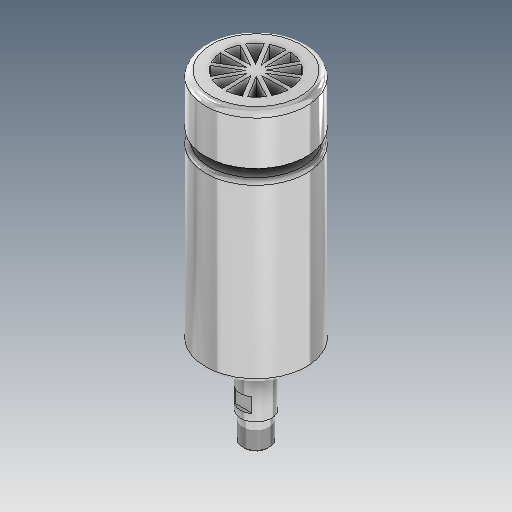
# Autodesk Inventor part: motor DC
Saved by Autodesk Inventor 2020 (Build 240168000, 168)
## iProperties
Created: 2020-05-03
Part Number: motor DC
Material: Genérico
Document SubType Name: Modeling
Designer: Leon
Density: 1 g/cm^3
Appearance: Cromo - Pulido
Mass: 286.743 g
Surface Area: 284.251 cm^2
Volume: 286.743 cm^3
Author: Leon
Autodesk Inventor part; units mm, degrees
ref_plane "YZ Plane" through (0, 0, 0) normal (1, 0, 0) x (0, 1, 0)
sketch "Boceto1" plane through (0, 0, 0) normal (0, 1, 0) x (-1, 0, 0)
  line L0 (66.6115, -79.4796) -> (66.6115, 152.1717)
  line L1 (66.6115, -79.4796) -> (92.6115, -79.4796)
  line L2 (92.6115, -79.4796) -> (92.6115, -53.9796)
  line L3 (92.6115, -53.9796) -> (79.6115, -53.9796)
  line L4 (79.6115, -53.9796) -> (79.6115, -48.4796)
  line L5 (79.6115, -48.4796) -> (92.6115, -48.4796)
  line L6 (92.6115, -48.4796) -> (92.6115, 41.8204)
  line L7 (92.6115, 41.8204) -> (79.6115, 41.8204)
  line L8 (79.6115, 41.8204) -> (79.6115, 48.3204)
  line L9 (79.6115, 48.3204) -> (70.6115, 48.3204)
  line L10 (70.6115, 48.3204) -> (70.6115, 51.8204)
  line L11 (70.6115, 51.8204) -> (74.6115, 51.8204)
  line L12 (74.6115, 51.8204) -> (74.6115, 71.8204)
  line L13 (74.6115, 71.8204) -> (73.5115, 71.8204)
  line L14 (73.5115, 71.8204) -> (73.5115, 86.3204)
  line L15 (73.5115, 86.3204) -> (66.6115, 86.3204)
  dimension "d8" = 26
  dimension "d9" = 25.5
  dimension "d10" = 13
  dimension "d11" = 5.5
  dimension "d12" = 90.3
  dimension "d20" = 13
  dimension "d21" = 6.5
  dimension "d22" = 9
  dimension "d23" = 3.5
  dimension "d24" = 4
  dimension "d25" = 20
  dimension "d26" = 1.1
  dimension "d27" = 14.5
  constraints: 32 end point, 10 perpendicular, 3 horizontal, 3 vertical, 2 point on line
  measures "d8" distance of L0.start L1.end
  measures "d9" distance of L1.end L2.end
  measures "d10" distance of L2.end L3.end
  measures "d11" distance of L3.end L4.end
  measures "d12" distance of L5.end L6.end
  measures "d20" distance of L6.end L7.end
  measures "d21" distance of L7.end L8.end
  measures "d22" distance of L8.end L9.end
  measures "d23" distance of L9.end L10.end
  measures "d24" distance of L10.end L11.end
  measures "d25" distance of L11.end L12.end
  measures "d26" distance of L12.end L13.end
  measures "d27" distance of L13.end L14.end
revolve "Revolución1" add sketch "Boceto1" angle 360 about axis through (-66.6115, 0, -79.4796) along (0, 0, 1)
fillet "Empalme1" radius 3 1 edges at (-40.6115, 0, -79.4796)
fillet "Empalme2" radius 2 1 edges at (-40.6115, 0, -48.4796)
fillet "Empalme3" radius 2 1 edges at (-40.6115, 0, 41.8204)
chamfer "Chaflán1" distance 1 angle 45 1 edges at (-59.7115, 0, 86.3204)
thread "Rosca1" size "M14x0.75" class "6g" standard "ISO Metric profile" length 9
sketch "Boceto3" plane through (-66.6115, 0, -79.4796) normal (0, 0, -1) x (-1, 0, 0)
  circle A0 centre (0, 0) radius 17
  line L0 (0, 0) -> (1, 0)
  line L1 (1, 0) -> (1, -16.9706)
  line L2 (0, 0) -> (-1, 0)
  line L3 (-1, 0) -> (-1, -16.9706)
  line L4 (0.866, 0.5) -> (9.3513, -14.1969)
  line L5 (-0.866, -0.5) -> (7.6193, -15.1969)
  line L6 (0.5, 0.866) -> (15.1969, -7.6193)
  line L7 (-0.5, -0.866) -> (14.1969, -9.3513)
  line L8 (0, 1) -> (16.9706, 1)
  line L9 (0, -1) -> (16.9706, -1)
  line L10 (-0.5, 0.866) -> (14.1969, 9.3513)
  line L11 (0.5, -0.866) -> (15.1969, 7.6193)
  line L12 (-0.866, 0.5) -> (7.6193, 15.1969)
  line L13 (0.866, -0.5) -> (9.3513, 14.1969)
  line L14 (-1, 0) -> (-1, 16.9706)
  line L15 (1, 0) -> (1, 16.9706)
  line L16 (-0.866, -0.5) -> (-9.3513, 14.1969)
  line L17 (0.866, 0.5) -> (-7.6193, 15.1969)
  line L18 (-0.5, -0.866) -> (-15.1969, 7.6193)
  line L19 (0.5, 0.866) -> (-14.1969, 9.3513)
  line L20 (0, -1) -> (-16.9706, -1)
  line L21 (0, 1) -> (-16.9706, 1)
  line L22 (0.5, -0.866) -> (-14.1969, -9.3513)
  line L23 (-0.5, 0.866) -> (-15.1969, -7.6193)
  line L24 (0.866, -0.5) -> (-7.6193, -15.1969)
  line L25 (-0.866, 0.5) -> (-9.3513, -14.1969)
  point P0 (-66.6115, 0)
  point P1 (9.3513, 14.1969)
  point P2 (2.7321, 2.7321)
  point P3 (1, 16.9706)
  point P4 (1, 3.7321)
  point P5 (7.6193, 15.1969)
  point P6 (-7.6193, 15.1969)
  point P7 (-1, 3.7321)
  point P8 (-1, 16.9706)
  point P9 (-2.7321, 2.7321)
  point P10 (-9.3513, 14.1969)
  point P11 (-3.7321, 1)
  point P12 (-15.1969, -7.6193)
  point P13 (-3.7321, -1)
  point P14 (-2.7321, -2.7321)
  point P15 (-1, -3.7321)
  point P16 (-7.6193, -15.1969)
  point P17 (7.6193, -15.1969)
  point P18 (1, -3.7321)
  point P19 (14.1969, -9.3513)
  point P20 (2.7321, -2.7321)
  point P21 (9.3513, -14.1969)
  point P22 (16.9706, -1)
  point P23 (3.7321, -1)
  point P24 (15.1969, -7.6193)
  point P25 (15.1969, 7.6193)
  point P26 (3.7321, 1)
  point P27 (16.9706, 1)
  dimension "d38" = 34
  dimension "d39" = 1
  dimension "d40" = 1
  dimension "d43" = 360
  constraints: 52 end point, 2 point on circle, 1 centre point, 1 horizontal, 1 perpendicular, 1 point on line, 73 other
  measures "d38" diameter of A0
  measures "d39" distance of L0.start L0.end
  measures "d40" distance of L0.start L2.end
extrude "Extrusión4" cut sketch "Boceto3" against normal blind 26 contours L8 L11 A0 | A0 L6 L9 | L10 L13 A0 | A0 L4 L7 | L12 L15 A0 | A0 L1 L5 | L14 L17 A0 | A0 L24 L3 | L16 L19 A0 | A0 L22 L25 | L18 L21 A0 | A0 L20 L23
ref_plane "Plano de trabajo1" through (-52.4146, 9.3513, -79.4796) normal (0.8784, -0.478, 0) x (0.478, 0.8784, 0)
sketch "Boceto4" plane through (-52.4146, 9.3513, -79.4796) normal (0.8784, -0.478, 0) x (0.478, 0.8784, 0)
  line L0 (-7, 151.3) -> (-7, 131.3) projected
  line L1 (-10.5, 147.8) -> (-19.5, 147.8)
  line L2 (-23, 151.3) -> (-23, 131.3) projected
  line L3 (-19.5, 140.3) -> (-10.5, 140.3)
  line L4 (-23, 151.3) -> (-7, 151.3) projected
  line L5 (-15, 140.3) -> (-19.5, 140.3)
  line L6 (-19.5, 140.3) -> (-10.5, 140.3)
  line L7 (-10.5, 140.3) -> (-10.5, 147.8)
  line L8 (-19.5, 140.3) -> (-19.5, 147.8)
  point P0 (16.8407, 79.4796)
  dimension "d49" = 3.5
  dimension "d50" = 4.5
  dimension "d51" = 9
  constraints: 12 end point, 2 perpendicular, 1 midpoint
  measures "d49" distance between parallel lines of L1 L4
  measures "d50" distance of L3.start L5.start
  measures "d51" distance of L3.start L3.end
extrude "Extrusión5" cut sketch "Boceto4" against normal blind 1.75
ref_plane "Plano de trabajo2" through (-80.8084, -9.3513, -79.4796) normal (-0.8784, 0.478, 0) x (-0.478, -0.8784, 0)
sketch "Boceto5" plane through (-80.8084, -9.3513, -79.4796) normal (-0.8784, 0.478, 0) x (-0.478, -0.8784, 0)
  line L0 (-23, 151.3) -> (-7, 151.3) projected
  line L1 (-7, 151.3) -> (-7, 131.3) projected
  line L2 (-19.5, 147.8) -> (-19.5, 140.3) projected
  line L3 (-19.5, 147.8) -> (-19.5, 140.3)
  line L4 (-19.5, 140.3) -> (-10.5, 140.3) projected
  line L5 (-19.5, 140.3) -> (-10.5, 140.3)
  line L6 (-10.5, 140.3) -> (-10.5, 147.8) projected
  line L7 (-10.5, 140.3) -> (-10.5, 147.8)
  line L8 (-10.5, 147.8) -> (-19.5, 147.8) projected
  line L9 (-10.5, 147.8) -> (-19.5, 147.8)
  circle A0 centre (-15, 135.5805) radius 1.75
  point P0 (-46.8407, 79.4796)
  dimension "d55" = 8
  dimension "d56" = 3.5
  constraints: 8 end point, 3 collinear, 1 centre point, 1 perpendicular
  measures "d55" distance from line of L1 A0.centre
  measures "d56" diameter of A0
extrude "Extrusión6" cut sketch "Boceto5" against normal blind 1.75 contours L8 L6 L4 L2
extrude "Extrusión7" cut sketch "Boceto5" against normal blind 4 contours A0
hole "Agujero1" at (-73.6384, 3.824, 56.1009) direction (0.8784, -0.478, 0) diameter 3.5 depth 4 tip angle 118
thread "Rosca2" size "M3.5x0.6" class "6H" standard "ISO Metric profile" length 9
sketch "Boceto6" plane through (-66.6115, 0, 86.3204) normal (0, 0, 1) x (1, 0, 0)
  circle A0 centre (0, 0) radius 5
  point P0 (66.6115, 0)
  dimension "d70" = 10
  constraints: 1 centre point
  measures "d70" diameter of A0
hole "Agujero2" at (-66.6115, 0, 86.3204) direction (0, 0, -1) diameter 10 depth 20 tip angle 118
